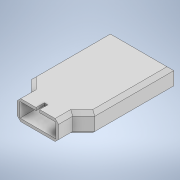
# Autodesk Inventor part: Cap
Saved by Autodesk Inventor 2021 (Build 250183000, 183)
## iProperties
Created: 2021-03-07
Part Number: Cap
Material: Generic
Document SubType Name: Modeling
Designer: mista
Density: 1 g/cm^3
Appearance: Default
Author: mista
Autodesk Inventor part; units mm, degrees
ref_plane "YZ Plane" through (0, 0, 0) normal (1, 0, 0) x (0, 1, 0)
ref_plane "XZ Plane" through (0, 0, 0) normal (0, 1, 0) x (-1, 0, 0)
ref_plane "XY Plane" through (0, 0, 0) normal (0, 0, 1) x (1, 0, 0)
sketch "Sketch1" plane through (0, 0, 0) normal (0, 0, 1) x (1, 0, 0)
  line L0 (0, 0) -> (33.274, 0)
  line L1 (33.274, 0) -> (33.274, 13.462)
  line L2 (33.274, 13.462) -> (0, 13.462)
  line L3 (0, 13.462) -> (0, 0)
  line L4 (-2.54, 16.002) -> (35.814, 16.002)
  line L5 (35.814, 16.002) -> (35.814, -2.54)
  line L6 (35.814, -2.54) -> (-2.54, -2.54)
  line L7 (-2.54, -2.54) -> (-2.54, 16.002)
  dimension "d0" = 33.274
  dimension "d1" = 13.462
  dimension "d2" = 2.54
  constraints: 16 end point, 4 parallel, 2 perpendicular, 1 horizontal, 3 other
  measures "d0" distance of L2.end L1.end
  measures "d1" distance of L1.end L0.end
  measures "d2" distance between parallel lines of L2 L4
extrude "Extrusion1" add sketch "Sketch1" against normal blind 13.208
sketch "Sketch3" plane through (0, 0, 0) normal (0, 0, 1) x (1, 0, 0)
  line L0 (14.986, 16.002) -> (14.986, 13.462)
  line L1 (0, 13.462) -> (33.274, 13.462)
  line L2 (35.814, 16.002) -> (-2.54, 16.002)
  line L3 (-2.54, 16.002) -> (-2.54, -2.54)
  line L4 (18.288, 16.002) -> (18.288, 13.462)
  line L5 (35.814, -2.54) -> (35.814, 16.002)
  line L6 (14.986, 16.002) -> (18.288, 16.002)
  line L7 (18.288, 13.462) -> (14.986, 13.462)
  line L8 (33.274, 13.462) -> (33.274, 0)
  line L9 (0, 0) -> (0, 13.462)
  dimension "d5" = 0
  dimension "d6" = 0
  dimension "d7" = 14.986
  dimension "d8" = 14.986
  constraints: 20 end point, 2 collinear, 1 parallel, 1 vertical
  measures "d5" distance from line of L1 L0.end
  measures "d6" distance from line of L2 L0.start
  measures "d7" distance between parallel lines of L8 L4
  measures "d8" distance between parallel lines of L0 L9
extrude "Extrusion2" cut sketch "Sketch3" against normal blind 7.62
sketch "Sketch4" plane through (0, 0, 0) normal (0, 1, 0) x (-1, 0, 0)
  line L0 (10.287, -23.368) -> (-43.561, -23.368)
  line L1 (-43.561, -23.368) -> (-43.561, -94.234)
  line L2 (-43.561, -94.234) -> (10.287, -94.234)
  line L3 (10.287, -94.234) -> (10.287, -23.368)
  circle A0 centre (-41.529, -25.4) radius 1.016
  circle A1 centre (8.255, -25.4) radius 1.016
  circle A2 centre (8.255, -92.202) radius 1.016
  circle A3 centre (-41.529, -92.202) radius 1.016
  line L4 (-33.274, -13.208) -> (0, -13.208) projected
  line L5 (-16.637, -13.208) -> (-16.637, -16.4825)
  point P0 (0, 0)
  dimension "d11" = 53.848
  dimension "d12" = 70.866
  dimension "d14" = 2.032
  dimension "d15" = 2.032
  dimension "d16" = 2.032
  dimension "d17" = 2.032
  dimension "d18" = 2.032
  dimension "d19" = 2.032
  dimension "d20" = 2.032
  dimension "d21" = 2.032
  dimension "d22" = 2.032
  dimension "d23" = 2.032
  dimension "d24" = 2.032
  dimension "d25" = 2.032
  dimension "d26" = 26.924
  dimension "d27" = 10.16
  constraints: 10 end point, 4 centre point, 2 parallel, 1 horizontal, 1 midpoint, 1 perpendicular, 1 vertical
  measures "d11" distance of L2.end L1.end
  measures "d12" distance of L1.end L0.end
  measures "d14" diameter of A0
  measures "d15" diameter of A1
  measures "d16" diameter of A2
  measures "d17" diameter of A3
  measures "d18" distance from line of L1 A3.centre
  measures "d19" distance from line of A3.centre L2
  measures "d20" distance from line of L1 A0.centre
  measures "d21" distance from line of L0 A0.centre
  measures "d22" distance from line of L3 A1.centre
  measures "d23" distance from line of L0 A1.centre
  measures "d24" distance from line of L2 A2.centre
  measures "d25" distance from line of L3 A2.centre
  measures "d26" distance between parallel lines of L5 L3
  measures "d27" distance between parallel lines of L4 L0
ref_plane "Work Plane1" through (0, 0, -23.368) normal (0, 0, -1) x (-1, 0, 0)
sketch "Sketch5" plane through (0, 0, -23.368) normal (0, 0, -1) x (-1, 0, 0)
  line L0 (10.287, 0) -> (-43.561, 0) projected
  line L1 (-43.561, 0) -> (10.287, 0)
  line L2 (10.287, 13.462) -> (10.287, 0)
  line L3 (10.287, 0) -> (-43.561, 0)
  line L4 (12.827, -2.54) -> (-46.101, -2.54)
  line L5 (-46.101, -2.54) -> (-46.101, 16.002)
  line L6 (-46.101, -2.54) -> (12.827, -2.54)
  line L7 (12.827, -2.54) -> (12.827, 16.002)
  line L8 (12.827, 16.002) -> (-46.101, 16.002)
  line L9 (-46.101, 16.002) -> (-46.101, -2.54)
  line L10 (10.287, 0) -> (-43.561, 0)
  line L11 (-43.561, 0) -> (-43.561, 13.462)
  line L12 (-43.561, 13.462) -> (10.287, 13.462)
  line L13 (10.287, 13.462) -> (10.287, 0)
  point P0 (0, 0)
  constraints: 26 end point, 4 parallel, 3 horizontal, 3 perpendicular
sketch "Sketch6" plane through (0, 0, -13.208) normal (0, 0, -1) x (-1, 0, 0)
  line L0 (-35.814, -2.54) -> (2.54, -2.54) projected
  line L1 (2.54, -2.54) -> (2.54, 16.002) projected
  line L2 (2.54, 16.002) -> (-35.814, 16.002) projected
  line L3 (-35.814, 16.002) -> (-35.814, -2.54) projected
  line L4 (0, 13.462) -> (0, 0) projected
  line L5 (0, 0) -> (-33.274, 0) projected
  line L6 (-33.274, 0) -> (-33.274, 13.462) projected
  line L7 (-33.274, 13.462) -> (0, 13.462) projected
extrude "Extrusion3" add sketch "Sketch5" along normal blind 73.406
sketch "Sketch7" plane through (0, 0, -23.368) normal (0, 0, 1) x (1, 0, 0)
  line L0 (46.101, 16.002) -> (46.101, -2.54) projected
  line L1 (-12.827, 16.002) -> (46.101, 16.002) projected
  line L2 (-12.827, -2.54) -> (-12.827, 16.002) projected
  line L3 (46.101, -2.54) -> (-12.827, -2.54) projected
  line L4 (43.561, 13.462) -> (-10.287, 13.462) projected
  line L5 (43.561, 0) -> (43.561, 13.462) projected
  line L6 (-10.287, 0) -> (43.561, 0) projected
  line L7 (-10.287, 13.462) -> (-10.287, 0) projected
  point P0 (0, 0)
sketch "Sketch8" plane through (0, 0, -23.368) normal (0, 0, 1) x (1, 0, 0)
  point P0 (0, 0)
sketch "Sketch9" plane through (0, 0, 0) normal (0, 1, 0) x (-1, 0, 0)
  line L0 (2.54, -13.208) -> (-35.814, -13.208) projected
  line L1 (12.827, -23.368) -> (2.54, -13.208)
  line L2 (2.54, -13.208) -> (-35.814, -13.208)
  line L3 (-45.8486, -23.368) -> (12.827, -23.368)
  line L4 (-35.814, 0) -> (-35.814, -13.208) projected
  line L5 (-46.101, -23.368) -> (12.827, -23.368) projected
  line L6 (-35.814, -13.208) -> (-46.101, -23.368)
  line L7 (-46.101, -23.368) -> (12.827, -23.368)
  point P0 (0, 0)
  constraints: 10 end point, 2 collinear, 1 parallel
extrude "Extrusion5" add sketch "Sketch9" against normal blind 2.54
sketch "Sketch11" plane through (0, 0, 0) normal (0, 1, 0) x (1, 0, 0)
  line L0 (33.274, 0) -> (0, 0) projected
  line L1 (33.274, 0) -> (33.274, 13.208) projected
  line L2 (35.814, 13.208) -> (33.274, 13.208) projected
  line L3 (35.814, 13.208) -> (46.101, 23.368) projected
  line L4 (43.561, 23.368) -> (46.101, 23.368) projected
  line L5 (43.561, 23.368) -> (43.561, 96.774) projected
  line L6 (-10.287, 96.774) -> (43.561, 96.774) projected
  line L7 (-10.287, 23.368) -> (-10.287, 96.774) projected
  line L8 (-12.827, 23.368) -> (-10.287, 23.368) projected
  line L9 (-12.827, 23.368) -> (-2.54, 13.208) projected
  line L10 (0, 13.208) -> (-2.54, 13.208) projected
  line L11 (0, 0) -> (0, 13.208) projected
  line L12 (-12.827, 23.368) -> (-2.54, 13.208) projected
  line L13 (-11.0421, 25.1752) -> (0, 14.2694)
  line L14 (0, 0) -> (0, 13.208) projected
  line L15 (0, 13.208) -> (0, 14.2694)
  line L16 (-10.287, 23.368) -> (-10.287, 96.774) projected
  line L17 (-10.287, 24.4294) -> (-10.287, 23.368)
  line L18 (-12.827, 23.368) -> (-10.287, 23.368) projected
  line L19 (-10.287, 23.368) -> (-12.827, 23.368)
  line L20 (-2.54, 0) -> (-2.54, 13.208) projected
  line L21 (-12.827, 23.368) -> (-2.54, 13.208)
  line L22 (-2.54, 13.208) -> (0, 13.208)
  line L23 (16.637, 13.208) -> (16.637, 17.9384)
  line L24 (46.101, 23.368) -> (43.561, 23.368)
  line L25 (46.101, 23.368) -> (35.814, 13.208)
  line L26 (44.3161, 25.1752) -> (33.274, 14.2694)
  line L27 (33.274, 13.208) -> (33.274, 14.2694)
  line L28 (43.561, 24.4294) -> (43.561, 23.368)
  line L29 (35.814, 13.208) -> (33.274, 13.208)
  point P0 (43.561, 24.4294)
  dimension "d40" = 2.54
  constraints: 26 end point, 3 point on line, 3 symmetric about line, 2 parallel, 2 vertical, 1 collinear, 1 perpendicular
  measures "d40" distance between parallel lines of L9 L13
extrude "Extrusion7" add sketch "Sketch11" along normal up to surface (13.462 mm away) contours L27 L26 L5 L4 L3 L2 | L10 L9 L8 L7 L13 L15
sketch "Sketch12" plane through (-12.827, 13.462, -23.368) normal (0, 1, 0) x (1, 0, 0)
  line L0 (58.928, 0) -> (55.3134, 0) projected
  line L1 (55.3134, 0) -> (46.101, -9.0986) projected
  line L2 (46.101, -9.0986) -> (46.101, -10.16) projected
  line L3 (48.641, -10.16) -> (46.101, -10.16) projected
  line L4 (48.641, -10.16) -> (58.928, 0) projected
  line L5 (3.6146, 0) -> (0, 0) projected
  line L6 (0, 0) -> (10.287, -10.16) projected
  line L7 (12.827, -10.16) -> (10.287, -10.16) projected
  line L8 (12.827, -10.16) -> (12.827, -9.0986) projected
  line L9 (12.827, -9.0986) -> (3.6146, 0) projected
  line L10 (12.827, -23.368) -> (12.827, -10.16) projected
  line L11 (12.827, -10.16) -> (46.101, -10.16)
  line L12 (55.3134, 0) -> (3.6146, 0) projected
  line L13 (55.3134, 0) -> (3.6146, 0)
  constraints: 4 end point, 1 collinear, 1 perpendicular
extrude "Extrusion8" add sketch "Sketch12" along normal blind 2.54
sketch "Sketch13" plane through (0, 0, 0) normal (0, 1, 0) x (1, 0, 0)
  line L0 (43.561, 94.234) -> (-10.287, 94.234) projected
  line L1 (46.101, 96.774) -> (-12.827, 96.774) projected
  line L2 (-10.287, 94.234) -> (43.561, 94.234)
  line L3 (43.561, 94.234) -> (43.561, 96.774)
  line L4 (43.561, 96.774) -> (-10.287, 96.774)
  line L5 (-10.287, 96.774) -> (-10.287, 94.234)
  point P0 (0, 0)
  point P1 (-10.287, 96.774)
  constraints: 8 end point, 2 parallel, 1 horizontal, 1 perpendicular, 1 point on line
extrude "Extrusion9" add sketch "Sketch13" along normal up to next
chamfer "Chamfer1" distance 3.175 angle 45 14 edges at (-12.827, 16.002, -60.071) (46.101, 16.002, -60.071) (46.101, -2.54, -60.071) (-12.827, -2.54, -60.071) (16.637, 16.002, -96.774) (16.637, -2.54, -96.774) (40.9575, 16.002, -18.288) (40.9575, -2.54, -18.288) (-7.6835, 16.002, -18.288) (-7.6835, -2.54, -18.288) (35.814, 16.002, -6.604) (35.814, -2.54, -6.604) (-2.54, 16.002, -6.604) (-2.54, -2.54, -6.604)
body "Solid1"
